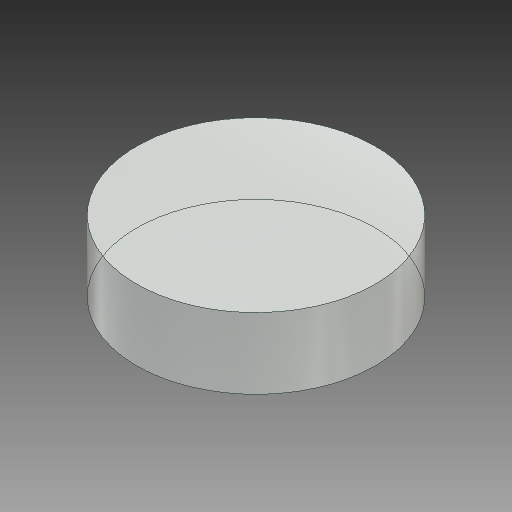
# Autodesk Inventor part: rotatingregion
Saved by Autodesk Inventor 2018 (Build 220112000, 112)
## iProperties
Created: 2018-02-05
Part Number: rotatingregion
Material: Glass
Document SubType Name: Modeling
Designer: Benedikt
Density: 2.18 g/cm^3
Appearance: Clear
Author: Benedikt
Autodesk Inventor part; units mm, degrees
ref_plane "YZ Plane" through (0, 0, 0) normal (1, 0, 0) x (0, 1, 0)
ref_plane "XZ Plane" through (0, 0, 0) normal (0, 1, 0) x (-1, 0, 0)
ref_plane "XY Plane" through (0, 0, 0) normal (0, 0, 1) x (1, 0, 0)
sketch "Sketch1" plane through (0, 0, 0) normal (0, 0, 1) x (1, 0, 0)
  circle A0 centre (0, 0) radius 43.8492
  dimension "d0" = 26
  constraints: 1 centre point, 1 coincident
extrude "Extrusion1" add sketch "Sketch1" against normal blind 26
body "Solid1"
